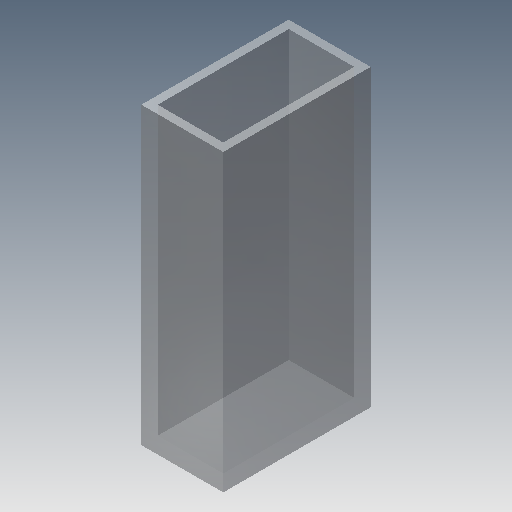
# Autodesk Inventor part: Küvette_20mm
Saved by Autodesk Inventor 2019 (Build 230136000, 136)
## iProperties
Created: 2015-10-07
Part Number: Küvette_20mm
Material: Glass
Document SubType Name: Modeling
Designer: voigt
Density: 2.18 g/cm^3
Appearance: Clear
Author: voigt
Autodesk Inventor part; units mm, degrees
ref_plane "YZ Plane" through (0, 0, 0) normal (1, 0, 0) x (0, 1, 0)
ref_plane "XZ Plane" through (0, 0, 0) normal (0, 1, 0) x (-1, 0, 0)
ref_plane "XY Plane" through (0, 0, 0) normal (0, 0, 1) x (1, 0, 0)
sketch "Sketch1" plane through (0, 0, 0) normal (0, 0, 1) x (1, 0, 0)
  line L0 (0, 15.75) -> (0, -15.75) construction
  line L1 (-8.75, 0) -> (8.75, 0) construction
  line L2 (-6.25, 11.25) -> (6.25, 11.25)
  line L3 (6.25, 11.25) -> (6.25, -11.25)
  line L4 (6.25, -11.25) -> (-6.25, -11.25)
  line L5 (-6.25, -11.25) -> (-6.25, 11.25)
  point P0 (0, 0)
  dimension "d0" = 22.5
  dimension "d1" = 12.5
  constraints: 8 end point, 2 parallel, 1 horizontal, 1 perpendicular, 2 other
  measures "d0" distance of L2.end L3.end
  measures "d1" distance of L3.end L4.end
extrude "Extrusion1" add sketch "Sketch1" along normal blind 45
sketch "Sketch2" plane through (0, 0, 45) normal (0, 0, 1) x (1, 0, 0)
  line L0 (-6.25, 11.25) -> (6.25, 11.25) projected
  line L1 (-6.25, -11.25) -> (-6.25, 11.25) projected
  line L2 (-5, 10) -> (5, 10)
  line L3 (5, 10) -> (5, -10)
  line L4 (5, -10) -> (-5, -10)
  line L5 (-5, -10) -> (-5, 10)
  point P0 (0, 0)
  dimension "d4" = 10
  dimension "d5" = 20
  dimension "d6" = 1.25
  dimension "d7" = 1.25
  constraints: 8 end point, 2 parallel, 1 horizontal, 1 perpendicular
  measures "d4" distance of L3.end L4.end
  measures "d5" distance of L2.end L3.end
  measures "d6" distance between parallel lines of L1 L5
  measures "d7" distance between parallel lines of L0 L2
extrude "Extrusion2" cut sketch "Sketch2" against normal blind 43.75
body "Solid1"
